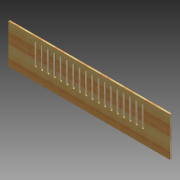
# Autodesk Inventor part: plywood back pannel 2
Saved by Autodesk Inventor 2012 (Build 160160000, 160)
## iProperties
Created: 2013-09-02
Part Number: plywood back pannel 2
Material: Default
Document SubType Name: Modeling
Designer: Bryce
Density: 1 g/cm^3
Author: Bryce
Autodesk Inventor part; units mm, degrees
ref_plane "YZ Plane" through (0, 0, 0) normal (1, 0, 0) x (0, 1, 0)
ref_plane "XZ Plane" through (0, 0, 0) normal (0, 1, 0) x (-1, 0, 0)
ref_plane "XY Plane" through (0, 0, 0) normal (0, 0, 1) x (1, 0, 0)
sketch "Sketch1" plane through (0, 0, 0) normal (0, 0, 1) x (1, 0, 0)
  line L0 (0, 0) -> (939.8, 0)
  line L1 (939.8, 0) -> (939.8, 228.6)
  line L2 (939.8, 228.6) -> (0, 228.6)
  line L3 (0, 228.6) -> (0, 0)
  line L4 (152.4, 76.2) -> (165.1, 76.2)
  line L5 (165.1, 76.2) -> (165.1, 203.2)
  line L6 (165.1, 203.2) -> (152.4, 203.2)
  line L7 (152.4, 203.2) -> (152.4, 76.2)
  line L8 (189.0065, 76.2) -> (201.7065, 76.2)
  line L9 (201.7065, 76.2) -> (201.7065, 203.2)
  line L10 (201.7065, 203.2) -> (189.0065, 203.2)
  line L11 (189.0065, 203.2) -> (189.0065, 76.2)
  line L12 (225.613, 76.2) -> (238.313, 76.2)
  line L13 (238.313, 76.2) -> (238.313, 203.2)
  line L14 (238.313, 203.2) -> (225.613, 203.2)
  line L15 (225.613, 203.2) -> (225.613, 76.2)
  line L16 (262.2194, 76.2) -> (274.9194, 76.2)
  line L17 (274.9194, 76.2) -> (274.9194, 203.2)
  line L18 (274.9194, 203.2) -> (262.2194, 203.2)
  line L19 (262.2194, 203.2) -> (262.2194, 76.2)
  line L20 (298.8259, 76.2) -> (311.5259, 76.2)
  line L21 (311.5259, 76.2) -> (311.5259, 203.2)
  line L22 (311.5259, 203.2) -> (298.8259, 203.2)
  line L23 (298.8259, 203.2) -> (298.8259, 76.2)
  line L24 (335.4324, 76.2) -> (348.1324, 76.2)
  line L25 (348.1324, 76.2) -> (348.1324, 203.2)
  line L26 (348.1324, 203.2) -> (335.4324, 203.2)
  line L27 (335.4324, 203.2) -> (335.4324, 76.2)
  line L28 (372.0389, 76.2) -> (384.7389, 76.2)
  line L29 (384.7389, 76.2) -> (384.7389, 203.2)
  line L30 (384.7389, 203.2) -> (372.0389, 203.2)
  line L31 (372.0389, 203.2) -> (372.0389, 76.2)
  line L32 (408.6454, 76.2) -> (421.3454, 76.2)
  line L33 (421.3454, 76.2) -> (421.3454, 203.2)
  line L34 (421.3454, 203.2) -> (408.6454, 203.2)
  line L35 (408.6454, 203.2) -> (408.6454, 76.2)
  line L36 (445.2518, 76.2) -> (457.9518, 76.2)
  line L37 (457.9518, 76.2) -> (457.9518, 203.2)
  line L38 (457.9518, 203.2) -> (445.2518, 203.2)
  line L39 (445.2518, 203.2) -> (445.2518, 76.2)
  line L40 (481.8583, 76.2) -> (494.5583, 76.2)
  line L41 (494.5583, 76.2) -> (494.5583, 203.2)
  line L42 (494.5583, 203.2) -> (481.8583, 203.2)
  line L43 (481.8583, 203.2) -> (481.8583, 76.2)
  line L44 (518.4648, 76.2) -> (531.1648, 76.2)
  line L45 (531.1648, 76.2) -> (531.1648, 203.2)
  line L46 (531.1648, 203.2) -> (518.4648, 203.2)
  line L47 (518.4648, 203.2) -> (518.4648, 76.2)
  line L48 (555.0713, 76.2) -> (567.7713, 76.2)
  line L49 (567.7713, 76.2) -> (567.7713, 203.2)
  line L50 (567.7713, 203.2) -> (555.0713, 203.2)
  line L51 (555.0713, 203.2) -> (555.0713, 76.2)
  line L52 (591.6778, 76.2) -> (604.3778, 76.2)
  line L53 (604.3778, 76.2) -> (604.3778, 203.2)
  line L54 (604.3778, 203.2) -> (591.6778, 203.2)
  line L55 (591.6778, 203.2) -> (591.6778, 76.2)
  line L56 (628.2842, 76.2) -> (640.9842, 76.2)
  line L57 (640.9842, 76.2) -> (640.9842, 203.2)
  line L58 (640.9842, 203.2) -> (628.2842, 203.2)
  line L59 (628.2842, 203.2) -> (628.2842, 76.2)
  line L60 (664.8907, 76.2) -> (677.5907, 76.2)
  line L61 (677.5907, 76.2) -> (677.5907, 203.2)
  line L62 (677.5907, 203.2) -> (664.8907, 203.2)
  line L63 (664.8907, 203.2) -> (664.8907, 76.2)
  line L64 (701.4972, 76.2) -> (714.1972, 76.2)
  line L65 (714.1972, 76.2) -> (714.1972, 203.2)
  line L66 (714.1972, 203.2) -> (701.4972, 203.2)
  line L67 (701.4972, 203.2) -> (701.4972, 76.2)
  line L68 (738.1037, 76.2) -> (750.8037, 76.2)
  line L69 (750.8037, 76.2) -> (750.8037, 203.2)
  line L70 (750.8037, 203.2) -> (738.1037, 203.2)
  line L71 (738.1037, 203.2) -> (738.1037, 76.2)
  line L72 (774.7102, 76.2) -> (787.4102, 76.2)
  line L73 (787.4102, 76.2) -> (787.4102, 203.2)
  line L74 (787.4102, 203.2) -> (774.7102, 203.2)
  line L75 (774.7102, 203.2) -> (774.7102, 76.2)
  dimension "d0" = 939.8
  dimension "d1" = 228.6
  dimension "d4" = 152.4
  dimension "d6" = 12.7
  dimension "d7" = 127
  dimension "d10" = 25.4
  dimension "d13" = 36.6065
  constraints: 152 end point, 4 parallel, 3 horizontal, 2 perpendicular, 136 other
  measures "d0" distance of L1.end L2.end
  measures "d1" distance of L2.end L0.start
  measures "d4" distance between parallel lines of L3 L7
  measures "d6" distance of L5.end L6.end
  measures "d7" distance of L6.end L4.start
  measures "d10" distance between parallel lines of L2 L6
  measures "d13" distance of L4.start L8.start
extrude "Extrusion1" add sketch "Sketch1" along normal blind 9.525
fillet "Fillet1" radius 6.35 72 edges at (165.1, 203.2, 4.7625) (152.4, 203.2, 4.7625) (152.4, 76.2, 4.7625) (165.1, 76.2, 4.7625) (787.4102, 76.2, 4.7625) (774.7102, 76.2, 4.7625) (750.8037, 76.2, 4.7625) (738.1037, 76.2, 4.7625) (714.1972, 76.2, 4.7625) (701.4972, 76.2, 4.7625) (677.5907, 76.2, 4.7625) (664.8907, 76.2, 4.7625) (640.9842, 76.2, 4.7625) (628.2842, 76.2, 4.7625) (604.3778, 76.2, 4.7625) (591.6778, 76.2, 4.7625) (567.7713, 76.2, 4.7625) (555.0713, 76.2, 4.7625) (531.1648, 76.2, 4.7625) (518.4648, 76.2, 4.7625) (494.5583, 76.2, 4.7625) (481.8583, 76.2, 4.7625) (457.9518, 76.2, 4.7625) (445.2518, 76.2, 4.7625) (421.3454, 76.2, 4.7625) (408.6454, 76.2, 4.7625) (384.7389, 76.2, 4.7625) (372.0389, 76.2, 4.7625) (348.1324, 76.2, 4.7625) (335.4324, 76.2, 4.7625) (311.5259, 76.2, 4.7625) (298.8259, 76.2, 4.7625) (274.9194, 76.2, 4.7625) (262.2194, 76.2, 4.7625) (238.313, 76.2, 4.7625) (225.613, 76.2, 4.7625) (201.7065, 76.2, 4.7625) (189.0065, 76.2, 4.7625) (787.4102, 203.2, 4.7625) (774.7102, 203.2, 4.7625) (750.8037, 203.2, 4.7625) (738.1037, 203.2, 4.7625) (714.1972, 203.2, 4.7625) (701.4972, 203.2, 4.7625) (677.5907, 203.2, 4.7625) (664.8907, 203.2, 4.7625) (640.9842, 203.2, 4.7625) (628.2842, 203.2, 4.7625) (604.3778, 203.2, 4.7625) (591.6778, 203.2, 4.7625) (567.7713, 203.2, 4.7625) (555.0713, 203.2, 4.7625) (531.1648, 203.2, 4.7625) (518.4648, 203.2, 4.7625) (494.5583, 203.2, 4.7625) (481.8583, 203.2, 4.7625) (457.9518, 203.2, 4.7625) (445.2518, 203.2, 4.7625) (421.3454, 203.2, 4.7625) (408.6454, 203.2, 4.7625) (384.7389, 203.2, 4.7625) (372.0389, 203.2, 4.7625) (348.1324, 203.2, 4.7625) (335.4324, 203.2, 4.7625) (311.5259, 203.2, 4.7625) (298.8259, 203.2, 4.7625) (274.9194, 203.2, 4.7625) (262.2194, 203.2, 4.7625) (238.313, 203.2, 4.7625) (225.613, 203.2, 4.7625) (201.7065, 203.2, 4.7625) (189.0065, 203.2, 4.7625)
body "Solid1"
